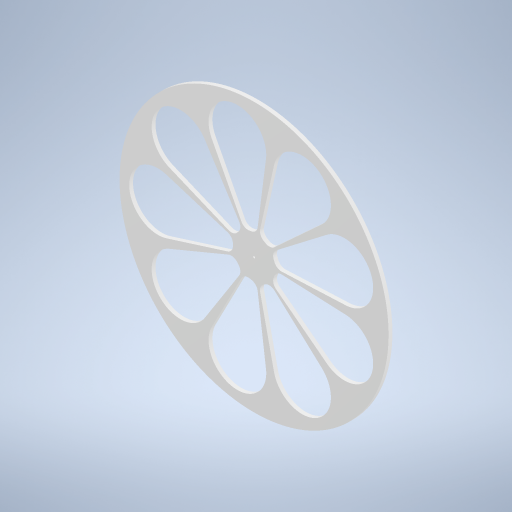
# Autodesk Inventor part: Backwheel
Saved by Autodesk Inventor 2023 (Build 270158000, 158)
## iProperties
Created: 2023-02-18
Part Number: Backwheel
Material: ABS Plastic
Document SubType Name: Modeling
Designer: phill
Density: 1.06 g/cm^3
Appearance: Smooth - White
Author: phill
Autodesk Inventor part; units mm, degrees
ref_plane "YZ Plane" through (0, 0, 0) normal (1, 0, 0) x (0, 1, 0)
ref_plane "Work Plane1" through (65.1894, 48.8955, 65.2669) normal (0, 0, 1) x (0, 1, 0)
ref_plane "Work Plane2" through (65.1894, 48.8955, 65.2669) normal (0, 0, 1) x (0, 1, 0)
sketch "Sketch2" plane through (65.1894, 48.8955, 65.2669) normal (0, 0, 1) x (0, 1, 0)
  circle A0 centre (0, 107) radius 1.5 projected
  arc A1 (217, 101.3826) -> (-3, 103.5) centre (-3, -11326.5) ccw projected
  line L0 (-3, 103.5) -> (-3, 110.5) projected
  arc A2 (-3, 110.5) -> (217, 112.6174) centre (-3, 11540.5) ccw projected
  line L1 (217, 112.6174) -> (217, 110) projected
  circle A3 centre (0, 107) radius 70
  circle A4 centre (0, 107) radius 0.5 projected
  circle A5 centre (0, 107) radius 1.5 projected
  line L2 (187, 104) -> (217, 104) projected
  line L3 (217, 104) -> (217, 101.3826) projected
  line L4 (217, 110) -> (187, 110) projected
  line L5 (187, 110) -> (187, 104) projected
  circle A6 centre (0, 107) radius 11
  circle A7 centre (0, 157) radius 15
  circle A8 centre (0, 107) radius 15
  line L6 (16.9932, 161.0351) -> (0, 107)
  line L7 (0, 107) -> (-16.6598, 159.9747)
  circle A9 centre (-32.1394, 145.3022) radius 15
  line L8 (-21.7155, 159.3163) -> (0, 107)
  line L9 (0, 107) -> (-46.8136, 136.8723)
  circle A10 centre (0, 107) radius 15
  circle A11 centre (0, 107) radius 11
  circle A12 centre (-49.2404, 115.6824) radius 15
  line L10 (-50.2633, 133.1182) -> (0, 107)
  line L11 (0, 107) -> (-55.0629, 99.7923)
  circle A13 centre (0, 107) radius 15
  circle A14 centre (0, 107) radius 11
  circle A15 centre (-43.3013, 82) radius 15
  line L12 (-55.2924, 94.699) -> (0, 107)
  line L13 (0, 107) -> (-37.5476, 66.0848)
  circle A16 centre (0, 107) radius 15
  circle A17 centre (0, 107) radius 11
  circle A18 centre (-17.101, 60.0154) radius 15
  line L14 (-34.4495, 62.0357) -> (0, 107)
  line L15 (0, 107) -> (-2.4634, 51.5221)
  circle A19 centre (0, 107) radius 15
  circle A20 centre (0, 107) radius 11
  circle A21 centre (17.101, 60.0154) radius 15
  line L16 (2.5127, 50.4116) -> (0, 107)
  line L17 (0, 107) -> (33.7735, 62.918)
  circle A22 centre (0, 107) radius 15
  circle A23 centre (0, 107) radius 11
  circle A24 centre (43.3013, 82) radius 15
  line L18 (38.2991, 65.2659) -> (0, 107)
  line L19 (0, 107) -> (54.2073, 94.9404)
  circle A25 centre (0, 107) radius 15
  circle A26 centre (0, 107) radius 11
  circle A27 centre (49.2404, 115.6824) radius 15
  line L20 (56.165, 99.648) -> (0, 107)
  line L21 (0, 107) -> (49.277, 132.6056)
  circle A28 centre (0, 107) radius 15
  circle A29 centre (0, 107) radius 11
  circle A30 centre (32.1394, 145.3022) radius 15
  line L22 (47.7506, 137.4702) -> (0, 107)
  line L23 (0, 107) -> (21.2894, 158.2897)
  circle A31 centre (0, 107) radius 15
  circle A32 centre (0, 107) radius 11
  point P0 (-48.8955, 65.1894)
  point P1 (9.2729, 112.9172)
  point P2 (4.217, 117.1596)
  point P3 (18.2854, 151.0527)
  point P4 (40.2082, 132.6573)
  point P5 (-4.217, 117.1596)
  point P6 (-9.2729, 112.9172)
  point P7 (-40.2082, 132.6573)
  point P8 (-18.2854, 151.0527)
  point P9 (7.4375, 98.8955)
  point P10 (10.4257, 103.4921)
  point P11 (15.8019, 103.4845)
  point P12 (46.5587, 96.642)
  point P13 (32.2496, 71.858)
  point P14 (9.7609, 112.072)
  point P15 (42.324, 128.9927)
  point P16 (57.7626, 103.3385)
  point P17 (27.0396, 103.4605)
  point P18 (10.907, 105.5723)
  point P19 (0.4879, 96.0108)
  point P20 (6.6899, 98.2682)
  point P21 (29.0081, 69.138)
  point P22 (2.1158, 59.35)
  point P23 (-6.6899, 98.2682)
  point P24 (-0.4879, 96.0108)
  point P25 (-2.1158, 59.35)
  point P26 (-29.0081, 69.138)
  point P27 (-10.7375, 104.6112)
  point P28 (-7.4375, 98.8955)
  point P29 (-32.2496, 71.858)
  point P30 (-46.5587, 96.642)
  point P31 (-9.7609, 112.072)
  point P32 (-10.907, 105.5723)
  point P33 (-47.2935, 100.8093)
  point P34 (-42.324, 128.9927)
  point P35 (-3.3, 117.4933)
  point P36 (-14.3091, 152.5)
  point P37 (14.3091, 152.5)
  point P38 (3.3, 117.4933)
  point P39 (10.7375, 104.6112)
  point P40 (47.2935, 100.8093)
  dimension "d0" = 140
  dimension "d3" = 22
  dimension "d4" = 30
  dimension "d7" = 50
  dimension "d8" = 4
  dimension "d11" = 360
  constraints: 36 end point, 28 centre point, 2 concentric, 2 tangent, 1 vertical alignment, 82 other
  measures "d0" diameter of A3
  measures "d3" diameter of A6
  measures "d4" diameter of A7
  measures "d7" distance of A3.centre A7.centre
  measures "d8" radial gap between concentric circles of A8 A6
extrude "Extrusion1" add sketch "Sketch2" along normal blind 2 contours A0 L20 A4 L21 | A0 L21 A2 A6 L20 | L21 A4 L22 A0 | A0 L22 A2 L21 | L20 A6 L19 A0 | A0 L19 A4 L20 | L22 A4 L23 A0 | A0 L23 A2 L22 | L21 A6 A2 | A2 L22 A6 L21 | L19 A6 A1 L18 A0 | A0 L18 A4 L19 | L20 A8 L19 A6 | L23 A4 L6 A0 | A0 L6 A2 L23 | A2 L23 A6 L22 | A6 L22 A8 L21 | L18 A1 L17 A0 | A0 L17 A4 L18 | L20 A1 L19 A8 | L6 A4 L7 A0 | A0 L7 A2 L6 | A2 L6 A6 L23 | A4 L8 A0 L7 | A4 L9 A0 L8 | A4 L10 A0 L9 | A4 L11 A0 L10 | A4 L12 A0 L11 | A4 L13 A0 L12 | A4 L14 A0 L13 | A4 L15 A0 L14 | A4 L16 A0 L15 | A4 L17 A0 L16 | A8 L22 A30 L23 L6 A7 L7 L8 A9 L9 L10 A12 L11 L12 A15 L13 L14 A18 L15 L16 A21 L17 L18 A24 L19 A1 L20 A27 A3 A2 L21 | L17 A1 L16 A0 | L18 A6 L17 A1 | A1 A6 L18 | A0 L8 A2 L7 | A2 L7 A6 L6 | A6 L6 A8 L23 | A0 L9 L0 A2 L8 | A0 L10 L0 L9 | A0 L11 L0 L10 | A0 L12 L0 L11 | A0 L13 L0 L12 | A0 L14 A1 L0 L13 | A0 L15 A1 L14 | A0 L16 A1 L15 | L17 A6 L16 A1 | L18 A8 L17 A6 | A2 L8 A6 L7 | A2 L0 L9 A6 L8 | L0 L10 A6 L9 | L0 L11 A6 L10 | L0 L12 A6 L11 | L0 L13 A6 L12 | L0 A1 L14 A6 L13 | A1 L15 A6 L14 | A1 L16 A6 L15 | A2 A3 A1 A27 | A6 L8 A8 L7 | A6 L10 A8 L9 | A6 L12 A8 L11 | A6 L14 A8 L13 | A6 L16 A8 L15
fillet "Fillet1" radius 4 18 edges at (-51.9701, 44.6784, 66.2669) (-47.7277, 39.6225, 66.2669) (-46.8826, 39.1346, 66.2669) (-39.4218, 38.158, 66.2669) (-40.3828, 37.9885, 66.2669) (-33.706, 41.458, 66.2669) (-30.8214, 48.4075, 66.2669) (-33.0787, 42.2055, 66.2669) (-30.8214, 49.3834, 66.2669) (-39.4218, 59.633, 66.2669) (-46.8826, 58.6563, 66.2669) (-33.0787, 55.5854, 66.2669) (-33.706, 56.333, 66.2669) (-40.3828, 59.8024, 66.2669) (-51.9701, 53.1125, 66.2669) (-52.3039, 45.5955, 66.2669) (-47.7277, 58.1684, 66.2669) (-52.3039, 52.1955, 66.2669)
body "Solid1"
